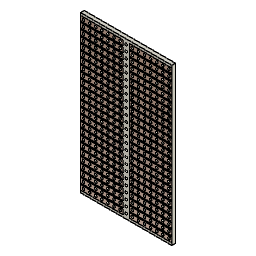
pcb_board (Autodesk Fusion 360 design; units mm, degrees)
Autodesk Fusion 360 part; units mm, degrees
sketch "Strip Board" plane through (0, 0, 0) normal (0, 1, 0) x (1, 0, 0)
  line L0 (0, 0) -> (38, 0)
  line L1 (38, 0) -> (38, -65)
  line L2 (38, -65) -> (0, -65)
  line L3 (0, -65) -> (0, 0)
  dimension "d3" = 38
  dimension "d4" = 65
  constraint horizontal L0
  constraint vertical L1
  constraint horizontal L2
  constraint vertical L3
  constraint coincident L0.start L3.end
  measures "d3" distance of L0.start L0.end
  measures "d4" distance of L0.end L1.end
extrude "Extrude1" add sketch "Strip Board" along normal blind 1.5 makes body 1
sketch "Holes" plane through (0, 0, 0) normal (0, -1, 0) x (1, 0, 0)
  line L0 (38, 65) -> (0, 65)
  line L1 (0, 65) -> (0, 0)
  line L2 (0, 0) -> (38, 0)
  line L3 (38, 0) -> (38, 65)
  circle A0 centre (1.22, 62.975) radius 0.5
  dimension "d5" = 1
  dimension "d12" = 1.22
  dimension "d13" = 2.025
  measures "d5" diameter of A0
  measures "d12" distance of L1 A0.centre
  measures "d13" distance of L0 A0.centre
extrude "Extrude2" cut sketch "Holes" against normal blind 1.5 contours A0 bodies 1
pattern_linear "R-Pattern1" count 25 spacing 2.5396 along (0, 0, -1) count 15 spacing 2.54 along (1, 0, 0) of "Extrude2"
sketch "Copper Strips" plane through (0, 0, 0) normal (0, -1, 0) x (1, 0, 0)
  circle A0 centre (36.78, 2.025) radius 0.5
  circle A1 centre (36.78, 4.5646) radius 0.5
  circle A2 centre (36.78, 7.1042) radius 0.5
  circle A3 centre (36.78, 9.6438) radius 0.5
  circle A4 centre (36.78, 12.1833) radius 0.5
  circle A5 centre (36.78, 14.7229) radius 0.5
  circle A6 centre (36.78, 17.2625) radius 0.5
  circle A7 centre (36.78, 19.8021) radius 0.5
  circle A8 centre (36.78, 22.3417) radius 0.5
  circle A9 centre (36.78, 24.8813) radius 0.5
  circle A10 centre (36.78, 27.4208) radius 0.5
  circle A11 centre (36.78, 29.9604) radius 0.5
  circle A12 centre (36.78, 32.5) radius 0.5
  circle A13 centre (36.78, 35.0396) radius 0.5
  circle A14 centre (36.78, 37.5792) radius 0.5
  circle A15 centre (36.78, 40.1187) radius 0.5
  circle A16 centre (36.78, 42.6583) radius 0.5
  circle A17 centre (36.78, 45.1979) radius 0.5
  circle A18 centre (36.78, 47.7375) radius 0.5
  circle A19 centre (36.78, 50.2771) radius 0.5
  circle A20 centre (36.78, 52.8167) radius 0.5
  circle A21 centre (36.78, 55.3563) radius 0.5
  circle A22 centre (36.78, 57.8958) radius 0.5
  circle A23 centre (36.78, 60.4354) radius 0.5
  circle A24 centre (36.78, 62.975) radius 0.5
  circle A25 centre (34.24, 2.025) radius 0.5
  circle A26 centre (34.24, 4.5646) radius 0.5
  circle A27 centre (34.24, 7.1042) radius 0.5
  circle A28 centre (34.24, 9.6438) radius 0.5
  circle A29 centre (34.24, 12.1833) radius 0.5
  circle A30 centre (34.24, 14.7229) radius 0.5
  circle A31 centre (34.24, 17.2625) radius 0.5
  circle A32 centre (34.24, 19.8021) radius 0.5
  circle A33 centre (34.24, 22.3417) radius 0.5
  circle A34 centre (34.24, 24.8813) radius 0.5
  circle A35 centre (34.24, 27.4208) radius 0.5
  circle A36 centre (34.24, 29.9604) radius 0.5
  circle A37 centre (34.24, 32.5) radius 0.5
  circle A38 centre (34.24, 35.0396) radius 0.5
  circle A39 centre (34.24, 37.5792) radius 0.5
  circle A40 centre (34.24, 40.1187) radius 0.5
  circle A41 centre (34.24, 42.6583) radius 0.5
  circle A42 centre (34.24, 45.1979) radius 0.5
  circle A43 centre (34.24, 47.7375) radius 0.5
  circle A44 centre (34.24, 50.2771) radius 0.5
  circle A45 centre (34.24, 52.8167) radius 0.5
  circle A46 centre (34.24, 55.3563) radius 0.5
  circle A47 centre (34.24, 57.8958) radius 0.5
  circle A48 centre (34.24, 60.4354) radius 0.5
  circle A49 centre (34.24, 62.975) radius 0.5
  circle A50 centre (31.7, 2.025) radius 0.5
  circle A51 centre (31.7, 4.5646) radius 0.5
  circle A52 centre (31.7, 7.1042) radius 0.5
  circle A53 centre (31.7, 9.6438) radius 0.5
  circle A54 centre (31.7, 12.1833) radius 0.5
  circle A55 centre (31.7, 14.7229) radius 0.5
  circle A56 centre (31.7, 17.2625) radius 0.5
  circle A57 centre (31.7, 19.8021) radius 0.5
  circle A58 centre (31.7, 22.3417) radius 0.5
  circle A59 centre (31.7, 24.8813) radius 0.5
  circle A60 centre (31.7, 27.4208) radius 0.5
  circle A61 centre (31.7, 29.9604) radius 0.5
  circle A62 centre (31.7, 32.5) radius 0.5
  circle A63 centre (31.7, 35.0396) radius 0.5
  circle A64 centre (31.7, 37.5792) radius 0.5
  circle A65 centre (31.7, 40.1187) radius 0.5
  circle A66 centre (31.7, 42.6583) radius 0.5
  circle A67 centre (31.7, 45.1979) radius 0.5
  circle A68 centre (31.7, 47.7375) radius 0.5
  circle A69 centre (31.7, 50.2771) radius 0.5
  circle A70 centre (31.7, 52.8167) radius 0.5
  circle A71 centre (31.7, 55.3563) radius 0.5
  circle A72 centre (31.7, 57.8958) radius 0.5
  circle A73 centre (31.7, 60.4354) radius 0.5
  circle A74 centre (31.7, 62.975) radius 0.5
  circle A75 centre (29.16, 2.025) radius 0.5
  circle A76 centre (29.16, 4.5646) radius 0.5
  circle A77 centre (29.16, 7.1042) radius 0.5
  circle A78 centre (29.16, 9.6438) radius 0.5
  circle A79 centre (29.16, 12.1833) radius 0.5
  circle A80 centre (29.16, 14.7229) radius 0.5
  circle A81 centre (29.16, 17.2625) radius 0.5
  circle A82 centre (29.16, 19.8021) radius 0.5
  circle A83 centre (29.16, 22.3417) radius 0.5
  circle A84 centre (29.16, 24.8813) radius 0.5
  circle A85 centre (29.16, 27.4208) radius 0.5
  circle A86 centre (29.16, 29.9604) radius 0.5
  circle A87 centre (29.16, 32.5) radius 0.5
  circle A88 centre (29.16, 35.0396) radius 0.5
  circle A89 centre (29.16, 37.5792) radius 0.5
  circle A90 centre (29.16, 40.1187) radius 0.5
  circle A91 centre (29.16, 42.6583) radius 0.5
  circle A92 centre (29.16, 45.1979) radius 0.5
  circle A93 centre (29.16, 47.7375) radius 0.5
  circle A94 centre (29.16, 50.2771) radius 0.5
  circle A95 centre (29.16, 52.8167) radius 0.5
  circle A96 centre (29.16, 55.3563) radius 0.5
  circle A97 centre (29.16, 57.8958) radius 0.5
  circle A98 centre (29.16, 60.4354) radius 0.5
  circle A99 centre (29.16, 62.975) radius 0.5
  circle A100 centre (26.62, 2.025) radius 0.5
  circle A101 centre (26.62, 4.5646) radius 0.5
  circle A102 centre (26.62, 7.1042) radius 0.5
  circle A103 centre (26.62, 9.6438) radius 0.5
  circle A104 centre (26.62, 12.1833) radius 0.5
  circle A105 centre (26.62, 14.7229) radius 0.5
  circle A106 centre (26.62, 17.2625) radius 0.5
  circle A107 centre (26.62, 19.8021) radius 0.5
  circle A108 centre (26.62, 22.3417) radius 0.5
  circle A109 centre (26.62, 24.8813) radius 0.5
  circle A110 centre (26.62, 27.4208) radius 0.5
  circle A111 centre (26.62, 29.9604) radius 0.5
  circle A112 centre (26.62, 32.5) radius 0.5
  circle A113 centre (26.62, 35.0396) radius 0.5
  circle A114 centre (26.62, 37.5792) radius 0.5
  circle A115 centre (26.62, 40.1187) radius 0.5
  circle A116 centre (26.62, 42.6583) radius 0.5
  circle A117 centre (26.62, 45.1979) radius 0.5
  circle A118 centre (26.62, 47.7375) radius 0.5
  circle A119 centre (26.62, 50.2771) radius 0.5
  circle A120 centre (26.62, 52.8167) radius 0.5
  circle A121 centre (26.62, 55.3563) radius 0.5
  circle A122 centre (26.62, 57.8958) radius 0.5
  circle A123 centre (26.62, 60.4354) radius 0.5
  circle A124 centre (26.62, 62.975) radius 0.5
  circle A125 centre (24.08, 2.025) radius 0.5
  circle A126 centre (24.08, 4.5646) radius 0.5
  circle A127 centre (24.08, 7.1042) radius 0.5
  circle A128 centre (24.08, 9.6438) radius 0.5
  circle A129 centre (24.08, 12.1833) radius 0.5
  circle A130 centre (24.08, 14.7229) radius 0.5
  circle A131 centre (24.08, 17.2625) radius 0.5
  circle A132 centre (24.08, 19.8021) radius 0.5
  circle A133 centre (24.08, 22.3417) radius 0.5
  circle A134 centre (24.08, 24.8813) radius 0.5
  circle A135 centre (24.08, 27.4208) radius 0.5
  circle A136 centre (24.08, 29.9604) radius 0.5
  circle A137 centre (24.08, 32.5) radius 0.5
  circle A138 centre (24.08, 35.0396) radius 0.5
  circle A139 centre (24.08, 37.5792) radius 0.5
  circle A140 centre (24.08, 40.1187) radius 0.5
  circle A141 centre (24.08, 42.6583) radius 0.5
  circle A142 centre (24.08, 45.1979) radius 0.5
  circle A143 centre (24.08, 47.7375) radius 0.5
  circle A144 centre (24.08, 50.2771) radius 0.5
  circle A145 centre (24.08, 52.8167) radius 0.5
  circle A146 centre (24.08, 55.3563) radius 0.5
  circle A147 centre (24.08, 57.8958) radius 0.5
  circle A148 centre (24.08, 60.4354) radius 0.5
  circle A149 centre (24.08, 62.975) radius 0.5
  circle A150 centre (21.54, 2.025) radius 0.5
  circle A151 centre (21.54, 4.5646) radius 0.5
  circle A152 centre (21.54, 7.1042) radius 0.5
  circle A153 centre (21.54, 9.6438) radius 0.5
  circle A154 centre (21.54, 12.1833) radius 0.5
  circle A155 centre (21.54, 14.7229) radius 0.5
  circle A156 centre (21.54, 17.2625) radius 0.5
  circle A157 centre (21.54, 19.8021) radius 0.5
  circle A158 centre (21.54, 22.3417) radius 0.5
  circle A159 centre (21.54, 24.8813) radius 0.5
  circle A160 centre (21.54, 27.4208) radius 0.5
  circle A161 centre (21.54, 29.9604) radius 0.5
  circle A162 centre (21.54, 32.5) radius 0.5
  circle A163 centre (21.54, 35.0396) radius 0.5
  circle A164 centre (21.54, 37.5792) radius 0.5
  circle A165 centre (21.54, 40.1187) radius 0.5
  circle A166 centre (21.54, 42.6583) radius 0.5
  circle A167 centre (21.54, 45.1979) radius 0.5
  circle A168 centre (21.54, 47.7375) radius 0.5
  circle A169 centre (21.54, 50.2771) radius 0.5
  circle A170 centre (21.54, 52.8167) radius 0.5
  circle A171 centre (21.54, 55.3563) radius 0.5
  circle A172 centre (21.54, 57.8958) radius 0.5
  circle A173 centre (21.54, 60.4354) radius 0.5
  circle A174 centre (21.54, 62.975) radius 0.5
  circle A175 centre (19, 2.025) radius 0.5
  circle A176 centre (19, 4.5646) radius 0.5
  circle A177 centre (19, 7.1042) radius 0.5
  circle A178 centre (19, 9.6438) radius 0.5
  circle A179 centre (19, 12.1833) radius 0.5
  circle A180 centre (19, 14.7229) radius 0.5
  circle A181 centre (19, 17.2625) radius 0.5
  circle A182 centre (19, 19.8021) radius 0.5
  circle A183 centre (19, 22.3417) radius 0.5
  circle A184 centre (19, 24.8813) radius 0.5
  circle A185 centre (19, 27.4208) radius 0.5
  circle A186 centre (19, 29.9604) radius 0.5
  circle A187 centre (19, 32.5) radius 0.5
  circle A188 centre (19, 35.0396) radius 0.5
  circle A189 centre (19, 37.5792) radius 0.5
  circle A190 centre (19, 40.1187) radius 0.5
  circle A191 centre (19, 42.6583) radius 0.5
  circle A192 centre (19, 45.1979) radius 0.5
  circle A193 centre (19, 47.7375) radius 0.5
  circle A194 centre (19, 50.2771) radius 0.5
  circle A195 centre (19, 52.8167) radius 0.5
  circle A196 centre (19, 55.3563) radius 0.5
  circle A197 centre (19, 57.8958) radius 0.5
  circle A198 centre (19, 60.4354) radius 0.5
  circle A199 centre (19, 62.975) radius 0.5
  circle A200 centre (16.46, 2.025) radius 0.5
  circle A201 centre (16.46, 4.5646) radius 0.5
  circle A202 centre (16.46, 7.1042) radius 0.5
  circle A203 centre (16.46, 9.6438) radius 0.5
  circle A204 centre (16.46, 12.1833) radius 0.5
  circle A205 centre (16.46, 14.7229) radius 0.5
  circle A206 centre (16.46, 17.2625) radius 0.5
  circle A207 centre (16.46, 19.8021) radius 0.5
  circle A208 centre (16.46, 22.3417) radius 0.5
  circle A209 centre (16.46, 24.8813) radius 0.5
  circle A210 centre (16.46, 27.4208) radius 0.5
  circle A211 centre (16.46, 29.9604) radius 0.5
  circle A212 centre (16.46, 32.5) radius 0.5
  circle A213 centre (16.46, 35.0396) radius 0.5
  circle A214 centre (16.46, 37.5792) radius 0.5
  circle A215 centre (16.46, 40.1187) radius 0.5
  circle A216 centre (16.46, 42.6583) radius 0.5
  circle A217 centre (16.46, 45.1979) radius 0.5
  circle A218 centre (16.46, 47.7375) radius 0.5
  circle A219 centre (16.46, 50.2771) radius 0.5
  circle A220 centre (16.46, 52.8167) radius 0.5
  circle A221 centre (16.46, 55.3563) radius 0.5
  circle A222 centre (16.46, 57.8958) radius 0.5
  circle A223 centre (16.46, 60.4354) radius 0.5
  circle A224 centre (16.46, 62.975) radius 0.5
  circle A225 centre (13.92, 2.025) radius 0.5
  circle A226 centre (13.92, 4.5646) radius 0.5
  circle A227 centre (13.92, 7.1042) radius 0.5
  circle A228 centre (13.92, 9.6438) radius 0.5
  circle A229 centre (13.92, 12.1833) radius 0.5
  circle A230 centre (13.92, 14.7229) radius 0.5
  circle A231 centre (13.92, 17.2625) radius 0.5
  circle A232 centre (13.92, 19.8021) radius 0.5
  circle A233 centre (13.92, 22.3417) radius 0.5
  circle A234 centre (13.92, 24.8813) radius 0.5
  circle A235 centre (13.92, 27.4208) radius 0.5
  circle A236 centre (13.92, 29.9604) radius 0.5
  circle A237 centre (13.92, 32.5) radius 0.5
  circle A238 centre (13.92, 35.0396) radius 0.5
  circle A239 centre (13.92, 37.5792) radius 0.5
  circle A240 centre (13.92, 40.1187) radius 0.5
  circle A241 centre (13.92, 42.6583) radius 0.5
  circle A242 centre (13.92, 45.1979) radius 0.5
  circle A243 centre (13.92, 47.7375) radius 0.5
  circle A244 centre (13.92, 50.2771) radius 0.5
  circle A245 centre (13.92, 52.8167) radius 0.5
  circle A246 centre (13.92, 55.3563) radius 0.5
  circle A247 centre (13.92, 57.8958) radius 0.5
  circle A248 centre (13.92, 60.4354) radius 0.5
  circle A249 centre (13.92, 62.975) radius 0.5
  circle A250 centre (11.38, 2.025) radius 0.5
  circle A251 centre (11.38, 4.5646) radius 0.5
  circle A252 centre (11.38, 7.1042) radius 0.5
  circle A253 centre (11.38, 9.6438) radius 0.5
  circle A254 centre (11.38, 12.1833) radius 0.5
  circle A255 centre (11.38, 14.7229) radius 0.5
  circle A256 centre (11.38, 17.2625) radius 0.5
  circle A257 centre (11.38, 19.8021) radius 0.5
  circle A258 centre (11.38, 22.3417) radius 0.5
  circle A259 centre (11.38, 24.8813) radius 0.5
  circle A260 centre (11.38, 27.4208) radius 0.5
  circle A261 centre (11.38, 29.9604) radius 0.5
  circle A262 centre (11.38, 32.5) radius 0.5
  circle A263 centre (11.38, 35.0396) radius 0.5
  circle A264 centre (11.38, 37.5792) radius 0.5
  circle A265 centre (11.38, 40.1187) radius 0.5
  circle A266 centre (11.38, 42.6583) radius 0.5
  circle A267 centre (11.38, 45.1979) radius 0.5
  circle A268 centre (11.38, 47.7375) radius 0.5
  circle A269 centre (11.38, 50.2771) radius 0.5
  circle A270 centre (11.38, 52.8167) radius 0.5
  circle A271 centre (11.38, 55.3563) radius 0.5
  circle A272 centre (11.38, 57.8958) radius 0.5
  circle A273 centre (11.38, 60.4354) radius 0.5
  circle A274 centre (11.38, 62.975) radius 0.5
  circle A275 centre (8.84, 2.025) radius 0.5
  circle A276 centre (8.84, 4.5646) radius 0.5
  circle A277 centre (8.84, 7.1042) radius 0.5
  circle A278 centre (8.84, 9.6438) radius 0.5
  circle A279 centre (8.84, 12.1833) radius 0.5
  circle A280 centre (8.84, 14.7229) radius 0.5
  circle A281 centre (8.84, 17.2625) radius 0.5
  circle A282 centre (8.84, 19.8021) radius 0.5
  circle A283 centre (8.84, 22.3417) radius 0.5
  circle A284 centre (8.84, 24.8813) radius 0.5
  circle A285 centre (8.84, 27.4208) radius 0.5
  circle A286 centre (8.84, 29.9604) radius 0.5
  circle A287 centre (8.84, 32.5) radius 0.5
  circle A288 centre (8.84, 35.0396) radius 0.5
  circle A289 centre (8.84, 37.5792) radius 0.5
  circle A290 centre (8.84, 40.1187) radius 0.5
  circle A291 centre (8.84, 42.6583) radius 0.5
  circle A292 centre (8.84, 45.1979) radius 0.5
  circle A293 centre (8.84, 47.7375) radius 0.5
  circle A294 centre (8.84, 50.2771) radius 0.5
  circle A295 centre (8.84, 52.8167) radius 0.5
  circle A296 centre (8.84, 55.3563) radius 0.5
  circle A297 centre (8.84, 57.8958) radius 0.5
  circle A298 centre (8.84, 60.4354) radius 0.5
  circle A299 centre (8.84, 62.975) radius 0.5
  circle A300 centre (6.3, 2.025) radius 0.5
  circle A301 centre (6.3, 4.5646) radius 0.5
  circle A302 centre (6.3, 7.1042) radius 0.5
  circle A303 centre (6.3, 9.6438) radius 0.5
  circle A304 centre (6.3, 12.1833) radius 0.5
  circle A305 centre (6.3, 14.7229) radius 0.5
  circle A306 centre (6.3, 17.2625) radius 0.5
  circle A307 centre (6.3, 19.8021) radius 0.5
  circle A308 centre (6.3, 22.3417) radius 0.5
  circle A309 centre (6.3, 24.8813) radius 0.5
  circle A310 centre (6.3, 27.4208) radius 0.5
  circle A311 centre (6.3, 29.9604) radius 0.5
  circle A312 centre (6.3, 32.5) radius 0.5
  circle A313 centre (6.3, 35.0396) radius 0.5
  circle A314 centre (6.3, 37.5792) radius 0.5
  circle A315 centre (6.3, 40.1187) radius 0.5
  circle A316 centre (6.3, 42.6583) radius 0.5
  circle A317 centre (6.3, 45.1979) radius 0.5
  circle A318 centre (6.3, 47.7375) radius 0.5
  circle A319 centre (6.3, 50.2771) radius 0.5
  circle A320 centre (6.3, 52.8167) radius 0.5
  circle A321 centre (6.3, 55.3563) radius 0.5
  circle A322 centre (6.3, 57.8958) radius 0.5
  circle A323 centre (6.3, 60.4354) radius 0.5
  circle A324 centre (6.3, 62.975) radius 0.5
  circle A325 centre (3.76, 2.025) radius 0.5
  circle A326 centre (3.76, 4.5646) radius 0.5
  circle A327 centre (3.76, 7.1042) radius 0.5
  circle A328 centre (3.76, 9.6438) radius 0.5
  circle A329 centre (3.76, 12.1833) radius 0.5
  circle A330 centre (3.76, 14.7229) radius 0.5
  circle A331 centre (3.76, 17.2625) radius 0.5
  circle A332 centre (3.76, 19.8021) radius 0.5
  circle A333 centre (3.76, 22.3417) radius 0.5
  circle A334 centre (3.76, 24.8813) radius 0.5
  circle A335 centre (3.76, 27.4208) radius 0.5
  circle A336 centre (3.76, 29.9604) radius 0.5
  circle A337 centre (3.76, 32.5) radius 0.5
  circle A338 centre (3.76, 35.0396) radius 0.5
  circle A339 centre (3.76, 37.5792) radius 0.5
  circle A340 centre (3.76, 40.1187) radius 0.5
  circle A341 centre (3.76, 42.6583) radius 0.5
  circle A342 centre (3.76, 45.1979) radius 0.5
  circle A343 centre (3.76, 47.7375) radius 0.5
  circle A344 centre (3.76, 50.2771) radius 0.5
  circle A345 centre (3.76, 52.8167) radius 0.5
  circle A346 centre (3.76, 55.3563) radius 0.5
  circle A347 centre (3.76, 57.8958) radius 0.5
  circle A348 centre (3.76, 60.4354) radius 0.5
  circle A349 centre (3.76, 62.975) radius 0.5
  circle A350 centre (1.22, 2.025) radius 0.5
  circle A351 centre (1.22, 4.5646) radius 0.5
  circle A352 centre (1.22, 7.1042) radius 0.5
  circle A353 centre (1.22, 9.6438) radius 0.5
  circle A354 centre (1.22, 12.1833) radius 0.5
  circle A355 centre (1.22, 14.7229) radius 0.5
  circle A356 centre (1.22, 17.2625) radius 0.5
  circle A357 centre (1.22, 19.8021) radius 0.5
  circle A358 centre (1.22, 22.3417) radius 0.5
  circle A359 centre (1.22, 24.8813) radius 0.5
  circle A360 centre (1.22, 27.4208) radius 0.5
  circle A361 centre (1.22, 29.9604) radius 0.5
  circle A362 centre (1.22, 32.5) radius 0.5
  circle A363 centre (1.22, 35.0396) radius 0.5
  circle A364 centre (1.22, 37.5792) radius 0.5
  circle A365 centre (1.22, 40.1187) radius 0.5
  circle A366 centre (1.22, 42.6583) radius 0.5
  circle A367 centre (1.22, 45.1979) radius 0.5
  circle A368 centre (1.22, 47.7375) radius 0.5
  circle A369 centre (1.22, 50.2771) radius 0.5
  circle A370 centre (1.22, 52.8167) radius 0.5
  circle A371 centre (1.22, 55.3563) radius 0.5
  circle A372 centre (1.22, 57.8958) radius 0.5
  circle A373 centre (1.22, 60.4354) radius 0.5
  circle A374 centre (1.22, 62.975) radius 0.5
  line L0 (38, 65) -> (0, 65)
  line L1 (0, 65) -> (0, 0)
  line L2 (0, 0) -> (38, 0)
  line L3 (38, 0) -> (38, 65)
  line L4 (0, 63.975) -> (38, 63.975)
  line L5 (38, 63.975) -> (38, 61.975)
  line L6 (38, 61.975) -> (0, 61.975)
  line L7 (0, 61.975) -> (0, 63.975)
  line L8 (38, 61.975) -> (0, 61.975)
  dimension "d14" = 2
  dimension "d15" = 1
  constraint horizontal L4
  constraint vertical L5
  constraint horizontal L6
  constraint vertical L7
  constraint coincident L1 L4.start
  constraint collinear L3 L5
  constraint horizontal L8
  measures "d14" distance of L4 L6
  measures "d15" distance of A374.centre L4
extrude "Extrude3" add sketch "Copper Strips" along normal blind 0.01 separate body contours L1 L3 L4 L5 L6 L7 L8 makes body 2
pattern_linear "R-Pattern2" count 25 spacing 2.5417 along (0, 0, -1) of bodies 2 makes body 3 at (0.24, 0, 60.4333) makes body 4 at (0.24, 0, 57.8917) makes body 5 at (0.24, 0, 55.35) makes body 6 at (0.24, 0, 52.8083) makes body 7 at (0.24, 0, 50.2667) makes body 8 at (0.24, 0, 47.725) makes body 9 at (0.24, 0, 45.1833) makes body 10 at (0.24, 0, 42.6417) makes body 11 at (0.24, 0, 40.1) makes body 12 at (0.24, 0, 37.5583) makes body 13 at (0.24, 0, 35.0167) makes body 14 at (0.24, 0, 32.475) makes body 15 at (0.24, 0, 29.9333) makes body 16 at (0.24, 0, 27.3917) makes body 17 at (0.24, 0, 24.85) makes body 18 at (0.24, 0, 22.3083) makes body 19 at (0.24, 0, 19.7667) makes body 20 at (0.24, 0, 17.225) makes body 21 at (0.24, 0, 14.6833) makes body 22 at (0.24, 0, 12.1417) makes body 23 at (0.24, 0, 9.6) makes body 24 at (0.24, 0, 7.0583) makes body 25 at (0.24, 0, 4.5167) makes body 26 at (0.24, 0, 1.975)
sketch "Middle Separator" plane through (0, -0.01, 0) normal (0, -1, 0) x (1, 0, 0)
  circle A0 centre (36.78, 62.975) radius 0.5
  circle A1 centre (31.7, 62.975) radius 0.5
  circle A2 centre (34.24, 62.975) radius 0.5
  circle A3 centre (29.16, 62.975) radius 0.5
  circle A4 centre (26.62, 62.975) radius 0.5
  circle A5 centre (24.08, 62.975) radius 0.5
  circle A6 centre (21.54, 62.975) radius 0.5
  circle A7 centre (13.92, 62.975) radius 0.5
  circle A8 centre (11.38, 62.975) radius 0.5
  circle A9 centre (8.84, 62.975) radius 0.5
  circle A10 centre (19, 62.975) radius 0.5
  circle A11 centre (16.46, 62.975) radius 0.5
  circle A12 centre (6.3, 62.975) radius 0.5
  circle A13 centre (3.76, 62.975) radius 0.5
  circle A14 centre (1.22, 62.975) radius 0.5
  line L0 (0, 61.975) -> (38, 61.975)
  line L1 (38, 61.975) -> (38, 63.975)
  line L2 (38, 63.975) -> (0, 63.975)
  line L3 (0, 63.975) -> (0, 61.975)
  line L4 (17.73, 65) -> (20.27, 65)
  line L5 (20.27, 65) -> (20.27, 0)
  line L6 (20.27, 0) -> (17.73, 0)
  line L7 (17.73, 0) -> (17.73, 65)
  line L8 (38, 65) -> (0, 65)
  line L9 (0, 0) -> (38, 0)
  dimension "d22" = 2.54
  dimension "d23" = 1.27
  constraint horizontal L4
  constraint vertical L5
  constraint horizontal L6
  constraint vertical L7
  constraint collinear L4 L8
  constraint collinear L6 L9
  measures "d22" distance of L5 L7
  measures "d23" distance of A10.centre L5
extrude "Extrude4" cut sketch "Middle Separator" against normal blind 0.01 contours L0 L2 L5 L7 | L0 L5 L6 L7 L9 | L2 L4 L5 L7 L8 bodies 2 3 4 5 6 7 8 9 10 11 12 13 14 15 16 17 18 19 20 21 22 23 24 25 26 makes body 51 at (17.4733, 0, 1.975) makes body 50 at (17.4733, 0, 4.5167) makes body 49 at (17.4733, 0, 7.0583) makes body 48 at (17.4733, 0, 9.6) makes body 47 at (17.4733, 0, 12.1417) makes body 46 at (17.4733, 0, 14.6833) makes body 45 at (17.4733, 0, 17.225) makes body 44 at (17.4733, 0, 19.7667) makes body 43 at (17.4733, 0, 22.3083) makes body 42 at (17.4733, 0, 24.85) makes body 41 at (17.4733, 0, 27.3917) makes body 40 at (17.4733, 0, 29.9333) makes body 39 at (17.4733, 0, 32.475) makes body 38 at (17.4733, 0, 35.0167) makes body 37 at (17.4733, 0, 37.5583) makes body 36 at (17.4733, 0, 40.1) makes body 35 at (17.4733, 0, 42.6417) makes body 34 at (17.4733, 0, 45.1833) makes body 33 at (17.4733, 0, 47.725) makes body 32 at (17.4733, 0, 50.2667) makes body 31 at (17.4733, 0, 52.8083) makes body 30 at (17.4733, 0, 55.35) makes body 29 at (17.4733, 0, 57.8917) makes body 28 at (17.4733, 0, 60.4333) makes body 27 at (17.4733, 0, 62.975)
equation "d12 = 0.72 mm + 0.5 mm"
equation "d13 = 1.525 mm + 0.5 mm"
equation "d23 = ( 2.54 / 2 ) * 1 mm"
named bodies: "Strip Board", "Copper Strip 1 Right", "Copper Strip 2 Right", "Copper Strip 3 Right", "Copper Strip 4 Right", "Copper Strip 5 Right", "Copper Strip 6 Right", "Copper Strip 7 Right", "Copper Strip 8 Right", "Copper Strip 9 Right", "Copper Strip 10 Right", "Copper Strip 11 Right", "Copper Strip 12 Right", "Copper Strip 13 Right", "Copper Strip 14 Right", "Copper Strip 15 Right", "Copper Strip 16 Right", "Copper Strip 17 Right", "Copper Strip 18 Right", "Copper Strip 19 Right", "Copper Strip 20 Right", "Copper Strip 21 Right", "Copper Strip 22 Right", "Copper Strip 23 Right", "Copper Strip 24 Right", "Copper Strip 25 Right", "Copper Strip 1 Left", "Copper Strip 2 Left", "Copper Strip 3 Left", "Copper Strip 4 Left", "Copper Strip 5 Left", "Copper Strip 6 Left", "Copper Strip 7 Left", "Copper Strip 8 Left", "Copper Strip 9 Left", "Copper Strip 10 Left", "Copper Strip 11 Left", "Copper Strip 12 Left", "Copper Strip 13 Left", "Copper Strip 14 Left", "Copper Strip 15 Left", "Copper Strip 16 Left", "Copper Strip 17 Left", "Copper Strip 18 Left", "Copper Strip 19 Left", "Copper Strip 20 Left", "Copper Strip 21 Left", "Copper Strip 22 Left", "Copper Strip 23 Left", "Copper Strip 24 Left", "Copper Strip 25 Left"
